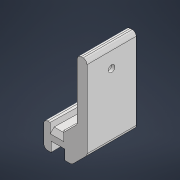
# Autodesk Inventor part: belt no touchy
Saved by Autodesk Inventor 2022 (Build 260153000, 153)
## iProperties
Created: 2022-02-10
Part Number: belt no touchy
Material: Generic
Document SubType Name: Modeling
Designer: nicol
Density: 1 g/cm^3
Appearance: Default
Author: nicol
Autodesk Inventor part; units mm, degrees
ref_plane "YZ Plane" through (0, 0, 0) normal (1, 0, 0) x (0, 1, 0)
ref_plane "XZ Plane" through (0, 0, 0) normal (0, 1, 0) x (-1, 0, 0)
ref_plane "XY Plane" through (0, 0, 0) normal (0, 0, 1) x (1, 0, 0)
sketch "Sketch1" plane through (0, 0, 0) normal (0, 0, 1) x (1, 0, 0)
  line L0 (0, 40.85) -> (0, 0)
  line L1 (0, 0) -> (-17, 0)
  line L2 (-17, 0) -> (-17, -5)
  line L3 (-17, -5) -> (5, -5)
  line L4 (5, -5) -> (5, 40.85)
  line L5 (5, 40.85) -> (0, 40.85)
  line L6 (-17, 0) -> (-17, 4)
  line L7 (-17, 4) -> (-15, 4)
  line L8 (-15, 4) -> (-15, 0)
  line L9 (-17, -5) -> (-17, -9)
  line L10 (-17, -9) -> (-15, -9)
  line L11 (-15, -9) -> (-15, -5)
  line L12 (-9, 0) -> (-9, 4)
  line L13 (-9, 4) -> (0, 4)
  line L14 (-9, -5) -> (-9, -9)
  line L15 (-9, -9) -> (5, -9)
  line L16 (5, -9) -> (5, -5)
  line L17 (-15, 4) -> (-9, 4)
  line L18 (-15, -9) -> (-9, -9)
  dimension "d0" = 5
  dimension "d1" = 15
  dimension "d2" = 4
  dimension "d3" = 2
  dimension "d4" = 40.85
  dimension "d5" = 6
  constraints: 38 end point, 9 perpendicular, 7 point on line, 4 vertical, 3 equal length, 3 horizontal, 2 collinear, 2 parallel, 1 coincident
  measures "d0" distance of L1.end L2.end
  measures "d1" distance between parallel lines of L0 L8
  measures "d2" distance of L7.end L8.end
  measures "d3" distance of L6.end L7.end
  measures "d4" distance between parallel lines of L5 L1
  measures "d5" distance between parallel lines of L8 L12
extrude "Extrusion1" add sketch "Sketch1" along normal blind 25
sketch "Sketch2" plane through (-17, 4, 0) normal (0, 1, 0) x (1, 0, 0)
  circle A0 centre (-1.4373, -213.5) radius 4.5 projected
  circle A1 centre (6.5, 197.5) radius 4.5 projected
  line L0 (10.8578, 8.8268) -> (10.0346, -33.8021)
  line L1 (10.0346, -33.8021) -> (3.0359, -33.667)
  line L2 (3.0359, -33.667) -> (3.8591, 8.9619)
  line L3 (3.8591, 8.9619) -> (10.8578, 8.8268)
  line L4 (3.0619, -213.5869) -> (10.9992, 197.4131)
  point P0 (17, 0)
  point P1 (6.5352, -33.7346)
  dimension "d8" = 7
  constraints: 10 end point, 3 perpendicular, 1 midpoint, 1 parallel, 1 point on line, 6 other
  measures "d8" distance between parallel lines of L2 L0
extrude "Extrusion2" cut sketch "Sketch2" against normal blind 3 contours L0 L1 L4 L3 | L4 L1 L2 L3
sketch "Sketch3" plane through (-17, -9, 0) normal (0, -1, 0) x (1, 0, 0)
  line L0 (3.2033, 25) -> (3.6861, 0) projected
  line L1 (10.6874, 0) -> (10.2046, 25) projected
  circle A0 centre (-1.4373, -188.5) radius 4.5 construction
  line L2 (22, 225.4393) -> (22, 219.5607) construction
  line L3 (22, 225.4393) -> (-378, 225.4393) construction
  line L4 (-378, 219.5607) -> (-378, 225.4393) construction
  line L5 (22, 219.5607) -> (-378, 219.5607) construction
  circle A1 centre (6.5, 222.5) radius 4.5 construction
  line L6 (3.0619, -188.5869) -> (10.9992, 222.4131) construction
  line L7 (11.0364, 43.0714) -> (4.0377, 43.2066)
  line L8 (4.0377, 43.2066) -> (2.5819, -32.1754)
  line L9 (2.5819, -32.1754) -> (9.5806, -32.3105)
  line L10 (9.5806, -32.3105) -> (11.0364, 43.0714)
  line L11 (3.6861, 0) -> (10.6874, 0) projected
  line L12 (10.2046, 25) -> (3.2033, 25) projected
  point P0 (17, 0)
  point P1 (7.537, 43.139)
  dimension "d38" = 7
  constraints: 10 end point, 3 parallel, 1 midpoint, 1 perpendicular, 1 point on line, 6 other
  measures "d38" distance between parallel lines of L8 L10
extrude "Extrusion3" cut sketch "Sketch3" against normal blind 3 contours L8 L12 L1 L10 L11 L0 | L0 L11 L10 L9 L8 | L8 L7 L10 L1 L12
chamfer "Chamfer1" distance 7.75 angle 45 1 edges at (5, -9, 12.5)
chamfer "Chamfer3" distance 6 angle 45 1 edges at (0, 4, 12.5)
sketch "Sketch5" plane through (0, 40.85, 0) normal (-1, 0, 0) x (0, 0, 1)
  line L0 (212.5, -7.0607) -> (212.5, -12.9393) projected
  line L1 (-187.5, -7.0607) -> (212.5, -7.0607) projected
  line L2 (-187.5, -12.9393) -> (-187.5, -7.0607) projected
  line L3 (-187.5, -12.9393) -> (212.5, -12.9393) projected
  line L4 (12.5, -7.0607) -> (12.5, -12.9393) construction
  line L5 (12.5, -10) -> (25, -10) construction
  line L6 (25, -42.1) -> (25, 0) projected
  line L7 (12.5, -10) -> (0, -10) construction
  line L8 (0, -42.1) -> (0, 0) projected
  point P0 (0, -40.85)
  constraints: 6 end point, 3 midpoint, 3 point on line, 1 coincident, 1 collinear, 1 horizontal, 1 vertical
hole "Hole1" at (0, 30.85, 12.5) direction (1, 0, 0) diameter 3.4 end through all counterbore diameter 6.5 counterbore depth 3.4 clearance for "Socket Head Cap Screw ISO 4762" size "M3" standard "ISO"
fillet "Fillet3" radius 2 7 edges at (-17, 4, 12.5) (-17, -9, 12.5) (-2.75, -9, 12.5) (5, -1.25, 12.5) (0, 10, 12.5) (5, 40.85, 12.5) (0, 40.85, 12.5)
chamfer "Chamfer4" distance 2 angle 45 4 edges at (-9.8133, 1, 0) (-10.2961, -6, 0) (-9.8133, -6, 25) (-10.2961, 1, 25)
body "Solid1"
